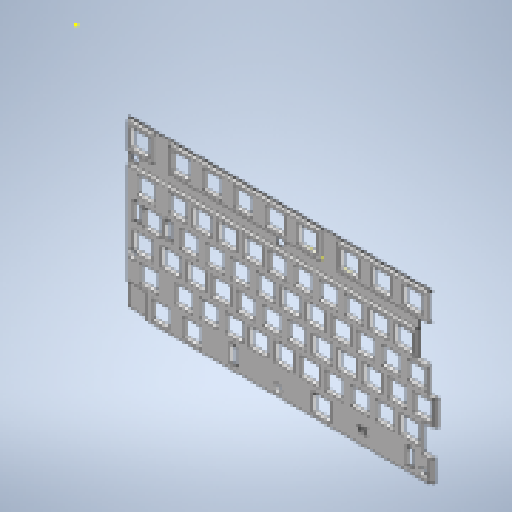
# Autodesk Inventor part: Left Plate
Saved by Autodesk Inventor 2025 (Build 290162000, 162)
## iProperties
Created: 2024-08-20
Part Number: Left Plate
Material: Generic
Document SubType Name: Modeling
Designer: adam
Density: 1 g/cm^3
Appearance: Default
Author: adam
Autodesk Inventor part; units mm, degrees
(part 1 of 2)
ref_plane "YZ Plane" through (0, 0, 0) normal (1, 0, 0) x (0, 1, 0)
ref_plane "XZ Plane" through (0, 0, 0) normal (0, 1, 0) x (-1, 0, 0)
ref_plane "XY Plane" through (0, 0, 0) normal (0, 0, 1) x (1, 0, 0)
sketch "Sketch2" plane through (0, 0, 0) normal (0, 0, 1) x (1, 0, 0)
  line L0 (490, -165) -> (40, -165) projected
  line L1 (490, -40) -> (490, -165) projected
  line L2 (40, -40) -> (490, -40) projected
  line L3 (40, -165) -> (40, -40) projected
  circle A0 centre (62.4608, -160.0704) radius 0.725 projected
  circle A1 centre (69.4608, -161.1204) radius 0.725 projected
  circle A2 centre (66.8608, -155.3704) radius 2.55 projected
  circle A3 centre (86.3368, -160.0704) radius 0.725 projected
  circle A4 centre (93.3368, -161.1204) radius 0.725 projected
  circle A5 centre (90.7368, -155.3704) radius 2.55 projected
  line L4 (118.6501, -160.3704) -> (124.6501, -160.3704) projected
  line L5 (118.6501, -145.3704) -> (118.6501, -160.3704) projected
  line L6 (124.6501, -145.3704) -> (118.6501, -145.3704) projected
  line L7 (124.6501, -160.3704) -> (124.6501, -145.3704) projected
  circle A6 centre (53.5708, -141.0204) radius 0.725 projected
  circle A7 centre (60.5708, -142.0704) radius 0.725 projected
  circle A8 centre (79.7328, -141.0204) radius 0.725 projected
  circle A9 centre (86.7328, -142.0704) radius 0.725 projected
  circle A10 centre (57.9708, -136.3204) radius 2.55 projected
  circle A11 centre (84.1328, -136.3204) radius 2.55 projected
  circle A12 centre (105.7828, -142.0704) radius 0.725 projected
  circle A13 centre (98.7828, -141.0204) radius 0.725 projected
  circle A14 centre (124.8328, -142.0704) radius 0.725 projected
  circle A15 centre (117.8328, -141.0204) radius 0.725 projected
  circle A16 centre (136.8828, -141.0204) radius 0.725 projected
  circle A17 centre (143.8828, -142.0704) radius 0.725 projected
  circle A18 centre (103.1828, -136.3204) radius 2.55 projected
  circle A19 centre (122.2328, -136.3204) radius 2.55 projected
  circle A20 centre (141.2828, -136.3204) radius 2.55 projected
  circle A21 centre (155, -160) radius 1.75 projected
  circle A22 centre (184.0001, -160.0704) radius 0.725 projected
  circle A23 centre (191.0001, -161.1204) radius 0.725 projected
  circle A24 centre (188.4001, -155.3704) radius 2.55 projected
  line L8 (252.1501, -160.3704) -> (258.1501, -160.3704) projected
  line L9 (252.1501, -145.3704) -> (252.1501, -160.3704) projected
  line L10 (258.1501, -145.3704) -> (252.1501, -145.3704) projected
  line L11 (258.1501, -160.3704) -> (258.1501, -145.3704) projected
  circle A25 centre (162.9328, -142.0704) radius 0.725 projected
  circle A26 centre (155.9328, -141.0204) radius 0.725 projected
  circle A27 centre (174.9828, -141.0204) radius 0.725 projected
  circle A28 centre (181.9828, -142.0704) radius 0.725 projected
  circle A29 centre (194.0328, -141.0204) radius 0.725 projected
  circle A30 centre (201.0328, -142.0704) radius 0.725 projected
  circle A31 centre (160.3328, -136.3204) radius 2.55 projected
  circle A32 centre (179.3828, -136.3204) radius 2.55 projected
  circle A33 centre (198.4328, -136.3204) radius 2.55 projected
  circle A34 centre (220.0828, -142.0704) radius 0.725 projected
  circle A35 centre (213.0828, -141.0204) radius 0.725 projected
  circle A36 centre (232.1368, -141.0224) radius 0.725 projected
  circle A37 centre (239.1368, -142.0724) radius 0.725 projected
  circle A38 centre (258.1768, -142.0924) radius 0.725 projected
  circle A39 centre (251.1768, -141.0424) radius 0.725 projected
  circle A40 centre (217.4828, -136.3204) radius 2.55 projected
  circle A41 centre (236.5368, -136.3224) radius 2.55 projected
  circle A42 centre (255.5768, -136.3424) radius 2.55 projected
  circle A43 centre (45, -127) radius 1.75 projected
  circle A44 centre (55.7448, -123.0204) radius 0.725 projected
  circle A45 centre (48.7448, -121.9704) radius 0.725 projected
  circle A46 centre (70.0808, -121.9704) radius 0.725 projected
  circle A47 centre (53.1448, -117.2704) radius 2.55 projected
  circle A48 centre (77.0808, -123.0204) radius 0.725 projected
  circle A49 centre (96.1308, -123.0204) radius 0.725 projected
  circle A50 centre (89.1308, -121.9704) radius 0.725 projected
  circle A51 centre (74.4808, -117.2704) radius 2.55 projected
  circle A52 centre (93.5308, -117.2704) radius 2.55 projected
  circle A53 centre (108.1808, -121.9704) radius 0.725 projected
  circle A54 centre (115.1808, -123.0204) radius 0.725 projected
  circle A55 centre (112.5808, -117.2704) radius 2.55 projected
  circle A56 centre (134.2308, -123.0204) radius 0.725 projected
  circle A57 centre (127.2308, -121.9704) radius 0.725 projected
  circle A58 centre (153.2808, -123.0204) radius 0.725 projected
  circle A59 centre (146.2808, -121.9704) radius 0.725 projected
  circle A60 centre (131.6308, -117.2704) radius 2.55 projected
  circle A61 centre (150.6808, -117.2704) radius 2.55 projected
  circle A62 centre (55.8568, -102.9204) radius 0.725 projected
  circle A63 centre (62.8568, -103.9704) radius 0.725 projected
  circle A64 centre (84.3048, -102.9204) radius 0.725 projected
  circle A65 centre (91.3048, -103.9704) radius 0.725 projected
  circle A66 centre (103.3548, -102.9204) radius 0.725 projected
  circle A67 centre (110.3548, -103.9704) radius 0.725 projected
  circle A68 centre (122.4048, -102.9204) radius 0.725 projected
  circle A69 centre (129.4048, -103.9704) radius 0.725 projected
  circle A70 centre (141.4548, -102.9204) radius 0.725 projected
  circle A71 centre (148.4548, -103.9704) radius 0.725 projected
  circle A72 centre (165.3308, -121.9704) radius 0.725 projected
  circle A73 centre (172.3308, -123.0204) radius 0.725 projected
  circle A74 centre (169.7308, -117.2704) radius 2.55 projected
  circle A75 centre (191.3808, -123.0204) radius 0.725 projected
  circle A76 centre (184.3808, -121.9704) radius 0.725 projected
  circle A77 centre (203.4308, -121.9704) radius 0.725 projected
  circle A78 centre (188.7808, -117.2704) radius 2.55 projected
  circle A79 centre (207.8308, -117.2704) radius 2.55 projected
  circle A80 centre (210.4308, -123.0204) radius 0.725 projected
  circle A81 centre (222.4808, -121.9704) radius 0.725 projected
  circle A82 centre (229.4808, -123.0204) radius 0.725 projected
  circle A83 centre (226.8808, -117.2704) radius 2.55 projected
  circle A84 centre (248.5308, -123.0204) radius 0.725 projected
  circle A85 centre (241.5308, -121.9704) radius 0.725 projected
  circle A86 centre (260.8348, -121.9704) radius 0.725 projected
  circle A87 centre (245.9308, -117.2704) radius 2.55 projected
  circle A88 centre (167.5048, -104.0492) radius 0.725 projected
  circle A89 centre (160.5048, -102.9992) radius 0.725 projected
  circle A90 centre (179.5548, -102.9204) radius 0.725 projected
  circle A91 centre (186.5548, -103.9704) radius 0.725 projected
  circle A92 centre (198.6048, -102.9204) radius 0.725 projected
  circle A93 centre (205.6048, -103.9704) radius 0.725 projected
  circle A94 centre (217.6548, -102.9204) radius 0.725 projected
  circle A95 centre (224.6548, -103.9704) radius 0.725 projected
  circle A96 centre (236.7048, -102.9204) radius 0.725 projected
  circle A97 centre (243.7048, -103.9704) radius 0.725 projected
  circle A98 centre (255.7548, -102.9204) radius 0.725 projected
  circle A99 centre (262.7548, -103.9704) radius 0.725 projected
  circle A100 centre (265, -160) radius 1.75 projected
  circle A101 centre (281.6628, -160.0704) radius 0.725 projected
  circle A102 centre (288.6628, -161.1204) radius 0.725 projected
  circle A103 centre (286.0628, -155.3704) radius 2.55 projected
  circle A104 centre (305.5388, -160.0704) radius 0.725 projected
  circle A105 centre (312.5388, -161.1204) radius 0.725 projected
  circle A106 centre (309.9388, -155.3704) radius 2.55 projected
  circle A107 centre (375, -160) radius 1.75 projected
  circle A108 centre (277.2328, -142.0704) radius 0.725 projected
  circle A109 centre (270.2328, -141.0204) radius 0.725 projected
  circle A110 centre (306.0468, -141.0204) radius 0.725 projected
  circle A111 centre (313.0468, -142.0704) radius 0.725 projected
  circle A112 centre (274.6328, -136.3204) radius 2.55 projected
  circle A113 centre (310.4468, -136.3204) radius 2.55 projected
  line L12 (295.4468, -141.3204) -> (301.4468, -141.3204) projected
  line L13 (295.4468, -126.3204) -> (295.4468, -141.3204) projected
  line L14 (301.4468, -126.3204) -> (295.4468, -126.3204) projected
  line L15 (301.4468, -141.3204) -> (301.4468, -126.3204) projected
  circle A114 centre (357.43, -142.0196) radius 0.725 projected
  circle A115 centre (350.43, -140.9696) radius 0.725 projected
  circle A116 centre (369.48, -140.9696) radius 0.725 projected
  line L16 (319.4468, -141.3204) -> (325.4468, -141.3204) projected
  line L17 (319.4468, -126.3204) -> (319.4468, -141.3204) projected
  line L18 (325.4468, -126.3204) -> (319.4468, -126.3204) projected
  line L19 (325.4468, -141.3204) -> (325.4468, -126.3204) projected
  circle A117 centre (354.83, -136.2696) radius 2.55 projected
  circle A118 centre (373.88, -136.2696) radius 2.55 projected
  circle A119 centre (426.8108, -160.0704) radius 0.725 projected
  circle A120 centre (431.2108, -155.3704) radius 2.55 projected
  line L20 (416.2108, -160.3704) -> (422.2108, -160.3704) projected
  line L21 (416.2108, -145.3704) -> (416.2108, -160.3704) projected
  line L22 (422.2108, -145.3704) -> (416.2108, -145.3704) projected
  line L23 (422.2108, -160.3704) -> (422.2108, -145.3704) projected
  circle A121 centre (433.8108, -161.1204) radius 0.725 projected
  circle A122 centre (455.2588, -160.0704) radius 0.725 projected
  circle A123 centre (462.2588, -161.1204) radius 0.725 projected
  circle A124 centre (459.6588, -155.3704) radius 2.55 projected
  line L24 (468.7088, -160.774) -> (483.7088, -160.774) projected
  line L25 (468.7088, -154.774) -> (468.7088, -160.774) projected
  line L26 (483.7088, -154.774) -> (468.7088, -154.774) projected
  line L27 (483.7088, -160.774) -> (483.7088, -154.774) projected
  line L28 (440.2108, -160.3704) -> (446.2108, -160.3704) projected
  line L29 (440.2108, -145.3704) -> (440.2108, -160.3704) projected
  line L30 (446.2108, -145.3704) -> (440.2108, -145.3704) projected
  line L31 (446.2108, -160.3704) -> (446.2108, -145.3704) projected
  circle A125 centre (483.4088, -150.174) radius 0.725 projected
  circle A126 centre (376.48, -142.0196) radius 0.725 projected
  circle A127 centre (388.53, -140.9696) radius 0.725 projected
  circle A128 centre (395.53, -142.0196) radius 0.725 projected
  circle A129 centre (417.1588, -140.922) radius 0.725 projected
  circle A130 centre (424.1588, -141.972) radius 0.725 projected
  circle A131 centre (392.93, -136.2696) radius 2.55 projected
  circle A132 centre (421.5588, -136.222) radius 2.55 projected
  circle A133 centre (443.2088, -141.972) radius 0.725 projected
  circle A134 centre (436.2088, -140.922) radius 0.725 projected
  circle A135 centre (455.2588, -140.922) radius 0.725 projected
  circle A136 centre (478.7088, -145.774) radius 2.55 projected
  circle A137 centre (462.2588, -141.972) radius 0.725 projected
  circle A138 centre (484.4588, -143.174) radius 0.725 projected
  circle A139 centre (440.6088, -136.222) radius 2.55 projected
  circle A140 centre (459.6588, -136.222) radius 2.55 projected
  line L32 (468.7088, -136.774) -> (483.7088, -136.774) projected
  line L33 (468.7088, -130.774) -> (468.7088, -136.774) projected
  line L34 (483.7088, -130.774) -> (468.7088, -130.774) projected
  line L35 (483.7088, -136.774) -> (483.7088, -130.774) projected
  circle A141 centre (267.8348, -123.0204) radius 0.725 projected
  circle A142 centre (286.8848, -123.0204) radius 0.725 projected
  circle A143 centre (279.8848, -121.9704) radius 0.725 projected
  circle A144 centre (265.2348, -117.2704) radius 2.55 projected
  circle A145 centre (284.2848, -117.2704) radius 2.55 projected
  circle A146 centre (305.9348, -123.0204) radius 0.725 projected
  circle A147 centre (298.9348, -121.9704) radius 0.725 projected
  circle A148 centre (303.3348, -117.2704) radius 2.55 projected
  line L36 (315.6708, -122.8724) -> (330.6708, -122.8724) projected
  line L37 (315.6708, -116.8724) -> (315.6708, -122.8724) projected
  line L38 (330.6708, -116.8724) -> (315.6708, -116.8724) projected
  line L39 (330.6708, -122.8724) -> (330.6708, -116.8724) projected
  circle A149 centre (369.48, -121.9196) radius 0.725 projected
  circle A150 centre (373.88, -117.2196) radius 2.55 projected
  circle A151 centre (274.8048, -102.9204) radius 0.725 projected
  circle A152 centre (281.8048, -103.9704) radius 0.725 projected
  circle A153 centre (293.8548, -102.9204) radius 0.725 projected
  circle A154 centre (300.8548, -103.9704) radius 0.725 projected
  circle A155 centre (329.3458, -112.2974) radius 0.725 projected
  circle A156 centre (324.6458, -107.8974) radius 2.55 projected
  circle A157 centre (330.3958, -105.2974) radius 0.725 projected
  circle A158 centre (376.48, -122.9696) radius 0.725 projected
  circle A159 centre (417.1588, -121.872) radius 0.725 projected
  circle A160 centre (424.1588, -122.922) radius 0.725 projected
  circle A161 centre (421.5588, -117.172) radius 2.55 projected
  circle A162 centre (485, -127) radius 1.75 projected
  circle A163 centre (443.2088, -122.922) radius 0.725 projected
  circle A164 centre (436.2088, -121.872) radius 0.725 projected
  circle A165 centre (455.2588, -121.872) radius 0.725 projected
  circle A166 centre (440.6088, -117.172) radius 2.55 projected
  circle A167 centre (462.2588, -122.922) radius 0.725 projected
  circle A168 centre (481.3088, -122.922) radius 0.725 projected
  circle A169 centre (474.3088, -121.872) radius 0.725 projected
  circle A170 centre (459.6588, -117.172) radius 2.55 projected
  circle A171 centre (478.7088, -117.172) radius 2.55 projected
  circle A172 centre (417.1588, -102.822) radius 0.725 projected
  circle A173 centre (424.1588, -103.872) radius 0.725 projected
  circle A174 centre (436.2088, -102.822) radius 0.725 projected
  circle A175 centre (443.2088, -103.872) radius 0.725 projected
  circle A176 centre (455.2588, -102.822) radius 0.725 projected
  circle A177 centre (462.2588, -103.872) radius 0.725 projected
  circle A178 centre (474.3088, -102.822) radius 0.725 projected
  circle A179 centre (481.3088, -103.872) radius 0.725 projected
  line L40 (45.2568, -103.2204) -> (51.2568, -103.2204) projected
  line L41 (45.2568, -88.2204) -> (45.2568, -103.2204) projected
  line L42 (51.2568, -88.2204) -> (45.2568, -88.2204) projected
  line L43 (51.2568, -103.2204) -> (51.2568, -88.2204) projected
  circle A180 centre (60.2568, -98.2204) radius 2.55 projected
  line L44 (69.2568, -103.2204) -> (75.2568, -103.2204) projected
  line L45 (69.2568, -88.2204) -> (69.2568, -103.2204) projected
  line L46 (75.2568, -88.2204) -> (69.2568, -88.2204) projected
  line L47 (75.2568, -103.2204) -> (75.2568, -88.2204) projected
  circle A181 centre (88.7048, -98.2204) radius 2.55 projected
  circle A182 centre (107.7548, -98.2204) radius 2.55 projected
  circle A183 centre (126.8048, -98.2204) radius 2.55 projected
  circle A184 centre (145.8548, -98.2204) radius 2.55 projected
  circle A185 centre (51.1288, -83.8704) radius 0.725 projected
  circle A186 centre (58.1288, -84.9204) radius 0.725 projected
  circle A187 centre (74.9068, -83.8704) radius 0.725 projected
  circle A188 centre (81.9068, -84.9204) radius 0.725 projected
  circle A189 centre (93.9568, -83.8704) radius 0.725 projected
  circle A190 centre (55.5288, -79.1704) radius 2.55 projected
  circle A191 centre (79.3068, -79.1704) radius 2.55 projected
  circle A192 centre (98.3568, -79.1704) radius 2.55 projected
  circle A193 centre (100.9568, -84.9204) radius 0.725 projected
  circle A194 centre (113.0068, -83.8704) radius 0.725 projected
  circle A195 centre (120.0068, -84.9204) radius 0.725 projected
  circle A196 centre (132.0568, -83.8704) radius 0.725 projected
  circle A197 centre (139.0568, -84.9204) radius 0.725 projected
  circle A198 centre (151.1068, -83.8704) radius 0.725 projected
  circle A199 centre (117.4068, -79.1704) radius 2.55 projected
  circle A200 centre (136.4568, -79.1704) radius 2.55 projected
  circle A201 centre (164.9048, -98.2992) radius 2.55 projected
  circle A202 centre (183.9548, -98.2204) radius 2.55 projected
  circle A203 centre (203.0048, -98.2204) radius 2.55 projected
  circle A204 centre (222.0548, -98.2204) radius 2.55 projected
  circle A205 centre (241.1048, -98.2204) radius 2.55 projected
  circle A206 centre (260.1548, -98.2204) radius 2.55 projected
  circle A207 centre (158.1068, -84.9204) radius 0.725 projected
  circle A208 centre (170.1568, -83.8704) radius 0.725 projected
  circle A209 centre (177.1568, -84.9204) radius 0.725 projected
  circle A210 centre (189.2068, -83.8704) radius 0.725 projected
  circle A211 centre (196.2068, -84.9204) radius 0.725 projected
  circle A212 centre (208.2568, -83.8704) radius 0.725 projected
  circle A213 centre (155.5068, -79.1704) radius 2.55 projected
  circle A214 centre (174.5568, -79.1704) radius 2.55 projected
  circle A215 centre (193.6068, -79.1704) radius 2.55 projected
  circle A216 centre (215.2568, -84.9204) radius 0.725 projected
  circle A217 centre (227.3068, -83.8704) radius 0.725 projected
  circle A218 centre (234.3068, -84.9204) radius 0.725 projected
  circle A219 centre (246.3568, -83.8704) radius 0.725 projected
  circle A220 centre (253.3568, -84.9204) radius 0.725 projected
  circle A221 centre (212.6568, -79.1704) radius 2.55 projected
  circle A222 centre (231.7068, -79.1704) radius 2.55 projected
  circle A223 centre (250.7568, -79.1704) radius 2.55 projected
  circle A224 centre (45, -64.8616) radius 1.75 projected
  circle A225 centre (50.8588, -50.6116) radius 2.55 projected
  circle A226 centre (81.9072, -50.3984) radius 2.55 projected
  circle A227 centre (48.2588, -44.8616) radius 0.725 projected
  circle A228 centre (55.2588, -45.9116) radius 0.725 projected
  circle A229 centre (79.3072, -44.6484) radius 0.725 projected
  circle A230 centre (86.3072, -45.6984) radius 0.725 projected
  circle A231 centre (105.7228, -50.5136) radius 2.55 projected
  circle A232 centre (129.5988, -50.5416) radius 2.55 projected
  circle A233 centre (153.4748, -50.5136) radius 2.55 projected
  circle A234 centre (103.1228, -44.7636) radius 0.725 projected
  circle A235 centre (110.1228, -45.8136) radius 0.725 projected
  circle A236 centre (126.9988, -44.7916) radius 0.725 projected
  circle A237 centre (133.9988, -45.8416) radius 0.725 projected
  circle A238 centre (150.8748, -44.7636) radius 0.725 projected
  circle A239 centre (155, -64.8616) radius 1.75 projected
  circle A240 centre (175.2648, -63.1601) radius 0.425 projected
  circle A241 centre (177.7648, -63.1601) radius 0.425 projected
  circle A242 centre (180.2648, -63.1601) radius 0.425 projected
  circle A243 centre (174.0148, -60.6601) radius 0.425 projected
  circle A244 centre (176.5148, -60.6601) radius 0.425 projected
  circle A245 centre (179.0148, -60.6601) radius 0.425 projected
  circle A246 centre (181.5148, -60.6601) radius 0.425 projected
  circle A247 centre (182.7648, -63.1601) radius 0.425 projected
  circle A248 centre (185.2648, -63.1601) radius 0.425 projected
  circle A249 centre (187.7648, -63.1601) radius 0.425 projected
  circle A250 centre (190.2648, -63.1601) radius 0.425 projected
  circle A251 centre (192.7648, -63.1601) radius 0.425 projected
  circle A252 centre (195.2648, -63.1601) radius 0.425 projected
  circle A253 centre (197.7648, -63.1601) radius 0.425 projected
  circle A254 centre (200.2648, -63.1601) radius 0.425 projected
  circle A255 centre (202.7648, -63.1601) radius 0.425 projected
  circle A256 centre (205.2648, -63.1601) radius 0.425 projected
  circle A257 centre (207.7648, -63.1601) radius 0.425 projected
  circle A258 centre (184.0148, -60.6601) radius 0.425 projected
  circle A259 centre (186.5148, -60.6601) radius 0.425 projected
  circle A260 centre (189.0148, -60.6601) radius 0.425 projected
  circle A261 centre (191.5148, -60.6601) radius 0.425 projected
  circle A262 centre (194.0148, -60.6601) radius 0.425 projected
  circle A263 centre (196.5148, -60.6601) radius 0.425 projected
  circle A264 centre (199.0148, -60.6601) radius 0.425 projected
  circle A265 centre (201.5148, -60.6601) radius 0.425 projected
  circle A266 centre (204.0148, -60.6601) radius 0.425 projected
  circle A267 centre (206.5148, -60.6601) radius 0.425 projected
  circle A268 centre (209.0148, -60.6601) radius 0.425 projected
  circle A269 centre (210.2648, -63.1601) radius 0.425 projected
  circle A270 centre (212.7648, -63.1601) radius 0.425 projected
  circle A271 centre (211.5148, -60.6601) radius 0.425 projected
  circle A272 centre (177.3508, -50.5136) radius 2.55 projected
  circle A273 centre (157.8748, -45.8136) radius 0.725 projected
  circle A274 centre (174.7508, -44.7636) radius 0.725 projected
  circle A275 centre (181.7508, -45.8136) radius 0.725 projected
  circle A276 centre (207.2568, -44.7636) radius 0.725 projected
  circle A277 centre (209.8568, -50.5136) radius 2.55 projected
  circle A278 centre (233.7388, -50.5136) radius 2.55 projected
  circle A279 centre (257.6148, -50.5136) radius 2.55 projected
  circle A280 centre (214.2568, -45.8136) radius 0.725 projected
  circle A281 centre (231.1388, -44.7636) radius 0.725 projected
  circle A282 centre (238.1388, -45.8136) radius 0.725 projected
  circle A283 centre (255.0148, -44.7636) radius 0.725 projected
  circle A284 centre (262.0148, -45.8136) radius 0.725 projected
  circle A285 centre (279.2048, -98.2204) radius 2.55 projected
  circle A286 centre (298.2548, -98.2204) radius 2.55 projected
  line L48 (315.6708, -98.8724) -> (330.6708, -98.8724) projected
  line L49 (315.6708, -92.8724) -> (315.6708, -98.8724) projected
  line L50 (330.6708, -92.8724) -> (315.6708, -92.8724) projected
  line L51 (330.6708, -98.8724) -> (330.6708, -92.8724) projected
  circle A287 centre (265.4068, -83.8704) radius 0.725 projected
  circle A288 centre (272.4068, -84.9204) radius 0.725 projected
  circle A289 centre (284.4568, -83.8704) radius 0.725 projected
  circle A290 centre (291.4568, -84.9204) radius 0.725 projected
  circle A291 centre (303.5068, -83.8704) radius 0.725 projected
  circle A292 centre (310.5068, -84.9204) radius 0.725 projected
  circle A293 centre (269.8068, -79.1704) radius 2.55 projected
  circle A294 centre (288.8568, -79.1704) radius 2.55 projected
  circle A295 centre (307.9068, -79.1704) radius 2.55 projected
  circle A296 centre (322.5568, -83.8704) radius 0.725 projected
  circle A297 centre (329.5568, -84.9204) radius 0.725 projected
  circle A298 centre (355.158, -83.8056) radius 0.725 projected
  circle A299 centre (362.158, -84.8556) radius 0.725 projected
  circle A300 centre (326.9568, -79.1704) radius 2.55 projected
  circle A301 centre (359.558, -79.1056) radius 2.55 projected
  circle A302 centre (421.5588, -98.122) radius 2.55 projected
  circle A303 centre (440.6088, -98.122) radius 2.55 projected
  circle A304 centre (459.6588, -98.122) radius 2.55 projected
  circle A305 centre (478.7088, -98.122) radius 2.55 projected
  circle A306 centre (383.754, -83.8056) radius 0.725 projected
  circle A307 centre (390.754, -84.8556) radius 0.725 projected
  circle A308 centre (417.1588, -83.772) radius 0.725 projected
  circle A309 centre (424.1588, -84.822) radius 0.725 projected
  circle A310 centre (388.154, -79.1056) radius 2.55 projected
  circle A311 centre (421.5588, -79.072) radius 2.55 projected
  circle A312 centre (436.2088, -83.772) radius 0.725 projected
  circle A313 centre (443.2088, -84.822) radius 0.725 projected
  circle A314 centre (455.2588, -83.772) radius 0.725 projected
  circle A315 centre (462.2588, -84.822) radius 0.725 projected
  circle A316 centre (474.3088, -83.772) radius 0.725 projected
  circle A317 centre (481.3088, -84.822) radius 0.725 projected
  circle A318 centre (440.6088, -79.072) radius 2.55 projected
  circle A319 centre (459.6588, -79.072) radius 2.55 projected
  circle A320 centre (478.7088, -79.072) radius 2.55 projected
  circle A321 centre (265, -64.8616) radius 1.75 projected
  circle A322 centre (375, -64.8616) radius 1.75 projected
  circle A323 centre (281.4908, -50.5136) radius 2.55 projected
  circle A324 centre (305.3668, -50.5136) radius 2.55 projected
  circle A325 centre (278.8908, -44.7636) radius 0.725 projected
  circle A326 centre (285.8908, -45.8136) radius 0.725 projected
  circle A327 centre (302.7668, -44.7636) radius 0.725 projected
  circle A328 centre (309.7668, -45.8136) radius 0.725 projected
  circle A329 centre (333.3668, -48.0136) radius 5 projected
  circle A330 centre (485, -64.8616) radius 1.75 projected
  circle A331 centre (408.3668, -48.0136) radius 5 projected
  circle A332 centre (453.2088, -50.322) radius 5 projected
  circle A333 centre (481.2088, -50.322) radius 5 projected
  circle A334 centre (432.68, -43) radius 0.5 projected
  circle A335 centre (435.22, -43) radius 0.5 projected
  circle A336 centre (437.76, -43) radius 0.5 projected
  circle A337 centre (440.3, -43) radius 0.5 projected
  line L52 (172.0148, -58.6601) -> (214.7648, -58.6601)
  line L53 (214.7648, -58.6601) -> (214.7648, -65.1601)
  line L54 (214.7648, -65.1601) -> (172.0148, -65.1601)
  line L55 (172.0148, -65.1601) -> (172.0148, -58.6601)
  line L56 (272.1064, -165) -> (272.1064, -148.1602) construction
  line L57 (272.1064, -148.1602) -> (265.1048, -148.1602) construction
  line L58 (265.1048, -148.1602) -> (265.1048, -126.7954) construction
  line L59 (265.1048, -126.7954) -> (274.7598, -126.7954) construction
  line L60 (274.7598, -126.7954) -> (274.7598, -107.7454) construction
  line L61 (274.7598, -107.7454) -> (269.6798, -107.7454) construction
  line L62 (269.6798, -107.7454) -> (269.6798, -88.6954) construction
  line L63 (269.6798, -88.6954) -> (260.2818, -88.6954) construction
  line L64 (260.2818, -88.6954) -> (260.2818, -61.0161) construction
  line L65 (260.2818, -61.0161) -> (269.5528, -61.0161) construction
  line L66 (269.5528, -61.0161) -> (269.5528, -40) construction
  line L67 (257.6148, -50.5136) -> (269.5528, -50.5136) construction
  line L68 (269.5528, -50.5136) -> (281.4908, -50.5136) construction
  line L69 (269.8068, -79.1704) -> (260.2818, -79.1704) construction
  line L70 (250.7568, -79.1704) -> (260.2818, -79.1704) construction
  line L71 (260.1548, -98.2204) -> (269.6798, -98.2204) construction
  line L72 (279.2048, -98.2204) -> (269.6798, -98.2204) construction
  line L73 (265.2348, -117.2704) -> (274.7598, -117.2704) construction
  line L74 (284.2848, -117.2704) -> (274.7598, -117.2704) construction
  line L75 (274.6328, -136.3204) -> (265.1048, -136.3204) construction
  line L76 (255.5768, -136.3424) -> (265.1048, -136.3204) construction
  line L77 (286.0628, -155.3704) -> (272.1064, -155.4026) construction
  line L78 (258.1501, -155.4349) -> (272.1064, -155.4026) construction
  line L79 (269.8688, -136.3204) -> (269.8688, -126.7954) construction
  line L80 (269.8688, -126.7954) -> (269.8688, -117.2704) construction
  line L81 (271.6818, -117.2704) -> (271.6818, -107.7454) construction
  line L82 (271.6818, -107.7454) -> (271.6818, -98.2204) construction
  line L83 (263.5838, -98.2204) -> (263.5838, -88.6954) construction
  line L84 (263.5838, -88.6954) -> (263.5838, -79.1704) construction
  line L85 (250.6123, -43.5111) -> (264.6173, -43.5111)
  line L86 (264.6173, -43.5111) -> (264.6173, -57.5161)
  line L87 (264.6173, -57.5161) -> (250.6123, -57.5161)
  line L88 (250.6123, -57.5161) -> (250.6123, -43.5111)
  line L89 (250.6123, -43.5111) -> (264.6173, -57.5161) construction
  line L90 (264.6173, -43.5111) -> (250.6123, -57.5161) construction
  line L91 (226.7363, -43.5111) -> (240.7413, -43.5111)
  line L92 (240.7413, -43.5111) -> (240.7413, -57.5161)
  line L93 (240.7413, -57.5161) -> (226.7363, -57.5161)
  line L94 (226.7363, -57.5161) -> (226.7363, -43.5111)
  line L95 (226.7363, -43.5111) -> (240.7413, -57.5161) construction
  line L96 (240.7413, -43.5111) -> (226.7363, -57.5161) construction
  line L97 (202.8543, -43.5111) -> (216.8593, -43.5111)
  line L98 (216.8593, -43.5111) -> (216.8593, -57.5161)
  line L99 (216.8593, -57.5161) -> (202.8543, -57.5161)
  line L100 (202.8543, -57.5161) -> (202.8543, -43.5111)
  line L101 (202.8543, -43.5111) -> (216.8593, -57.5161) construction
  line L102 (216.8593, -43.5111) -> (202.8543, -57.5161) construction
  line L103 (170.3483, -43.5111) -> (184.3533, -43.5111)
  line L104 (184.3533, -43.5111) -> (184.3533, -57.5161)
  line L105 (184.3533, -57.5161) -> (170.3483, -57.5161)
  line L106 (170.3483, -57.5161) -> (170.3483, -43.5111)
  line L107 (170.3483, -43.5111) -> (184.3533, -57.5161) construction
  line L108 (184.3533, -43.5111) -> (170.3483, -57.5161) construction
  line L109 (146.4723, -43.5111) -> (160.4773, -43.5111)
  line L110 (160.4773, -43.5111) -> (160.4773, -57.5161)
  line L111 (160.4773, -57.5161) -> (146.4723, -57.5161)
  line L112 (146.4723, -57.5161) -> (146.4723, -43.5111)
  line L113 (146.4723, -43.5111) -> (160.4773, -57.5161) construction
  line L114 (160.4773, -43.5111) -> (146.4723, -57.5161) construction
  line L115 (122.5963, -43.5391) -> (136.6013, -43.5391)
  line L116 (136.6013, -43.5391) -> (136.6013, -57.5441)
  line L117 (136.6013, -57.5441) -> (122.5963, -57.5441)
  line L118 (122.5963, -57.5441) -> (122.5963, -43.5391)
  line L119 (122.5963, -43.5391) -> (136.6013, -57.5441) construction
  line L120 (136.6013, -43.5391) -> (122.5963, -57.5441) construction
  line L121 (98.7203, -43.5111) -> (112.7253, -43.5111)
  line L122 (112.7253, -43.5111) -> (112.7253, -57.5161)
  line L123 (112.7253, -57.5161) -> (98.7203, -57.5161)
  line L124 (98.7203, -57.5161) -> (98.7203, -43.5111)
  line L125 (98.7203, -43.5111) -> (112.7253, -57.5161) construction
  line L126 (112.7253, -43.5111) -> (98.7203, -57.5161) construction
  line L127 (74.9047, -43.3959) -> (88.9097, -43.3959)
  line L128 (88.9097, -43.3959) -> (88.9097, -57.4009)
  line L129 (88.9097, -57.4009) -> (74.9047, -57.4009)
  line L130 (74.9047, -57.4009) -> (74.9047, -43.3959)
  line L131 (74.9047, -43.3959) -> (88.9097, -57.4009) construction
  line L132 (88.9097, -43.3959) -> (74.9047, -57.4009) construction
  line L133 (43.8563, -43.6091) -> (57.8613, -43.6091)
  line L134 (57.8613, -43.6091) -> (57.8613, -57.6141)
  line L135 (57.8613, -57.6141) -> (43.8563, -57.6141)
  line L136 (43.8563, -57.6141) -> (43.8563, -43.6091)
  line L137 (43.8563, -43.6091) -> (57.8613, -57.6141) construction
  line L138 (57.8613, -43.6091) -> (43.8563, -57.6141) construction
  line L139 (48.5263, -72.1679) -> (62.5313, -72.1679)
  line L140 (62.5313, -72.1679) -> (62.5313, -86.1729)
  line L141 (62.5313, -86.1729) -> (48.5263, -86.1729)
  line L142 (48.5263, -86.1729) -> (48.5263, -72.1679)
  line L143 (48.5263, -72.1679) -> (62.5313, -86.1729) construction
  line L144 (62.5313, -72.1679) -> (48.5263, -86.1729) construction
  line L145 (72.3043, -72.1679) -> (86.3093, -72.1679)
  line L146 (86.3093, -72.1679) -> (86.3093, -86.1729)
  line L147 (86.3093, -86.1729) -> (72.3043, -86.1729)
  line L148 (72.3043, -86.1729) -> (72.3043, -72.1679)
  line L149 (72.3043, -72.1679) -> (86.3093, -86.1729) construction
  line L150 (86.3093, -72.1679) -> (72.3043, -86.1729) construction
  line L151 (91.3543, -72.1679) -> (105.3593, -72.1679)
  line L152 (105.3593, -72.1679) -> (105.3593, -86.1729)
  line L153 (105.3593, -86.1729) -> (91.3543, -86.1729)
  line L154 (91.3543, -86.1729) -> (91.3543, -72.1679)
  line L155 (91.3543, -72.1679) -> (105.3593, -86.1729) construction
  line L156 (105.3593, -72.1679) -> (91.3543, -86.1729) construction
  line L157 (110.4043, -72.1679) -> (124.4093, -72.1679)
  line L158 (124.4093, -72.1679) -> (124.4093, -86.1729)
  line L159 (124.4093, -86.1729) -> (110.4043, -86.1729)
  line L160 (110.4043, -86.1729) -> (110.4043, -72.1679)
  line L161 (110.4043, -72.1679) -> (124.4093, -86.1729) construction
  line L162 (124.4093, -72.1679) -> (110.4043, -86.1729) construction
  line L163 (129.4543, -72.1679) -> (143.4593, -72.1679)
  line L164 (143.4593, -72.1679) -> (143.4593, -86.1729)
  line L165 (143.4593, -86.1729) -> (129.4543, -86.1729)
  line L166 (129.4543, -86.1729) -> (129.4543, -72.1679)
  line L167 (129.4543, -72.1679) -> (143.4593, -86.1729) construction
  line L168 (143.4593, -72.1679) -> (129.4543, -86.1729) construction
  line L169 (148.5043, -72.1679) -> (162.5093, -72.1679)
  line L170 (162.5093, -72.1679) -> (162.5093, -86.1729)
  line L171 (162.5093, -86.1729) -> (148.5043, -86.1729)
  line L172 (148.5043, -86.1729) -> (148.5043, -72.1679)
  line L173 (148.5043, -72.1679) -> (162.5093, -86.1729) construction
  line L174 (162.5093, -72.1679) -> (148.5043, -86.1729) construction
  line L175 (167.5543, -72.1679) -> (181.5593, -72.1679)
  line L176 (181.5593, -72.1679) -> (181.5593, -86.1729)
  line L177 (181.5593, -86.1729) -> (167.5543, -86.1729)
  line L178 (167.5543, -86.1729) -> (167.5543, -72.1679)
  line L179 (167.5543, -72.1679) -> (181.5593, -86.1729) construction
  line L180 (181.5593, -72.1679) -> (167.5543, -86.1729) construction
  line L181 (53.2543, -91.2179) -> (67.2593, -91.2179)
  line L182 (67.2593, -91.2179) -> (67.2593, -105.2229)
  line L183 (67.2593, -105.2229) -> (53.2543, -105.2229)
  line L184 (53.2543, -105.2229) -> (53.2543, -91.2179)
  line L185 (53.2543, -91.2179) -> (67.2593, -105.2229) construction
  line L186 (67.2593, -91.2179) -> (53.2543, -105.2229) construction
  line L187 (186.6043, -72.1679) -> (200.6093, -72.1679)
  line L188 (200.6093, -72.1679) -> (200.6093, -86.1729)
  line L189 (200.6093, -86.1729) -> (186.6043, -86.1729)
  line L190 (186.6043, -86.1729) -> (186.6043, -72.1679)
  line L191 (186.6043, -72.1679) -> (200.6093, -86.1729) construction
  line L192 (200.6093, -72.1679) -> (186.6043, -86.1729) construction
  line L193 (205.6543, -72.1679) -> (219.6593, -72.1679)
  line L194 (219.6593, -72.1679) -> (219.6593, -86.1729)
  line L195 (219.6593, -86.1729) -> (205.6543, -86.1729)
  line L196 (205.6543, -86.1729) -> (205.6543, -72.1679)
  line L197 (205.6543, -72.1679) -> (219.6593, -86.1729) construction
  line L198 (219.6593, -72.1679) -> (205.6543, -86.1729) construction
  line L199 (224.7043, -72.1679) -> (238.7093, -72.1679)
  line L200 (238.7093, -72.1679) -> (238.7093, -86.1729)
  line L201 (238.7093, -86.1729) -> (224.7043, -86.1729)
  line L202 (224.7043, -86.1729) -> (224.7043, -72.1679)
  line L203 (224.7043, -72.1679) -> (238.7093, -86.1729) construction
  line L204 (238.7093, -72.1679) -> (224.7043, -86.1729) construction
  line L205 (243.7543, -72.1679) -> (257.7593, -72.1679)
  line L206 (257.7593, -72.1679) -> (257.7593, -86.1729)
  line L207 (257.7593, -86.1729) -> (243.7543, -86.1729)
  line L208 (243.7543, -86.1729) -> (243.7543, -72.1679)
  line L209 (243.7543, -72.1679) -> (257.7593, -86.1729) construction
  line L210 (257.7593, -72.1679) -> (243.7543, -86.1729) construction
  line L211 (253.1523, -91.2179) -> (267.1573, -91.2179)
  line L212 (267.1573, -91.2179) -> (267.1573, -105.2229)
  line L213 (267.1573, -105.2229) -> (253.1523, -105.2229)
  line L214 (253.1523, -105.2229) -> (253.1523, -91.2179)
  line L215 (253.1523, -91.2179) -> (267.1573, -105.2229) construction
  line L216 (267.1573, -91.2179) -> (253.1523, -105.2229) construction
  line L217 (234.1023, -91.2179) -> (248.1073, -91.2179)
  line L218 (248.1073, -91.2179) -> (248.1073, -105.2229)
  line L219 (248.1073, -105.2229) -> (234.1023, -105.2229)
  line L220 (234.1023, -105.2229) -> (234.1023, -91.2179)
  line L221 (234.1023, -91.2179) -> (248.1073, -105.2229) construction
  line L222 (248.1073, -91.2179) -> (234.1023, -105.2229) construction
  line L223 (215.0523, -91.2179) -> (229.0573, -91.2179)
  line L224 (229.0573, -91.2179) -> (229.0573, -105.2229)
  line L225 (229.0573, -105.2229) -> (215.0523, -105.2229)
  line L226 (215.0523, -105.2229) -> (215.0523, -91.2179)
  line L227 (215.0523, -91.2179) -> (229.0573, -105.2229) construction
  line L228 (229.0573, -91.2179) -> (215.0523, -105.2229) construction
  line L229 (196.0023, -91.2179) -> (210.0073, -91.2179)
  line L230 (210.0073, -91.2179) -> (210.0073, -105.2229)
  line L231 (210.0073, -105.2229) -> (196.0023, -105.2229)
  line L232 (196.0023, -105.2229) -> (196.0023, -91.2179)
  line L233 (196.0023, -91.2179) -> (210.0073, -105.2229) construction
  line L234 (210.0073, -91.2179) -> (196.0023, -105.2229) construction
  line L235 (176.9523, -91.2179) -> (190.9573, -91.2179)
  line L236 (190.9573, -91.2179) -> (190.9573, -105.2229)
  line L237 (190.9573, -105.2229) -> (176.9523, -105.2229)
  line L238 (176.9523, -105.2229) -> (176.9523, -91.2179)
  line L239 (176.9523, -91.2179) -> (190.9573, -105.2229) construction
  line L240 (190.9573, -91.2179) -> (176.9523, -105.2229) construction
  line L241 (157.9023, -91.2967) -> (171.9073, -91.2967)
  line L242 (171.9073, -91.2967) -> (171.9073, -105.3017)
  line L243 (171.9073, -105.3017) -> (157.9023, -105.3017)
  line L244 (157.9023, -105.3017) -> (157.9023, -91.2967)
  line L245 (157.9023, -91.2967) -> (171.9073, -105.3017) construction
  line L246 (171.9073, -91.2967) -> (157.9023, -105.3017) construction
  line L247 (138.8523, -91.2179) -> (152.8573, -91.2179)
  line L248 (152.8573, -91.2179) -> (152.8573, -105.2229)
  line L249 (152.8573, -105.2229) -> (138.8523, -105.2229)
  line L250 (138.8523, -105.2229) -> (138.8523, -91.2179)
  line L251 (138.8523, -91.2179) -> (152.8573, -105.2229) construction
  line L252 (152.8573, -91.2179) -> (138.8523, -105.2229) construction
  line L253 (119.8023, -91.2179) -> (133.8073, -91.2179)
  line L254 (133.8073, -91.2179) -> (133.8073, -105.2229)
  line L255 (133.8073, -105.2229) -> (119.8023, -105.2229)
  line L256 (119.8023, -105.2229) -> (119.8023, -91.2179)
  line L257 (119.8023, -91.2179) -> (133.8073, -105.2229) construction
  line L258 (133.8073, -91.2179) -> (119.8023, -105.2229) construction
  line L259 (100.7523, -91.2179) -> (114.7573, -91.2179)
  line L260 (114.7573, -91.2179) -> (114.7573, -105.2229)
  line L261 (114.7573, -105.2229) -> (100.7523, -105.2229)
  line L262 (100.7523, -105.2229) -> (100.7523, -91.2179)
  line L263 (100.7523, -91.2179) -> (114.7573, -105.2229) construction
  line L264 (114.7573, -91.2179) -> (100.7523, -105.2229) construction
  line L265 (81.7023, -91.2179) -> (95.7073, -91.2179)
  line L266 (95.7073, -91.2179) -> (95.7073, -105.2229)
  line L267 (95.7073, -105.2229) -> (81.7023, -105.2229)
  line L268 (81.7023, -105.2229) -> (81.7023, -91.2179)
  line L269 (81.7023, -91.2179) -> (95.7073, -105.2229) construction
  line L270 (95.7073, -91.2179) -> (81.7023, -105.2229) construction
  line L271 (46.1423, -110.2679) -> (60.1473, -110.2679)
  line L272 (60.1473, -110.2679) -> (60.1473, -124.2729)
  line L273 (60.1473, -124.2729) -> (46.1423, -124.2729)
  line L274 (46.1423, -124.2729) -> (46.1423, -110.2679)
  line L275 (46.1423, -110.2679) -> (60.1473, -124.2729) construction
  line L276 (60.1473, -110.2679) -> (46.1423, -124.2729) construction
  line L277 (67.4783, -110.2679) -> (81.4833, -110.2679)
  line L278 (81.4833, -110.2679) -> (81.4833, -124.2729)
  line L279 (81.4833, -124.2729) -> (67.4783, -124.2729)
  line L280 (67.4783, -124.2729) -> (67.4783, -110.2679)
  line L281 (67.4783, -110.2679) -> (81.4833, -124.2729) construction
  line L282 (81.4833, -110.2679) -> (67.4783, -124.2729) construction
  line L283 (86.5283, -110.2679) -> (100.5333, -110.2679)
  line L284 (100.5333, -110.2679) -> (100.5333, -124.2729)
  line L285 (100.5333, -124.2729) -> (86.5283, -124.2729)
  line L286 (86.5283, -124.2729) -> (86.5283, -110.2679)
  line L287 (86.5283, -110.2679) -> (100.5333, -124.2729) construction
  line L288 (100.5333, -110.2679) -> (86.5283, -124.2729) construction
  line L289 (105.5783, -110.2679) -> (119.5833, -110.2679)
  line L290 (119.5833, -110.2679) -> (119.5833, -124.2729)
  line L291 (119.5833, -124.2729) -> (105.5783, -124.2729)
  line L292 (105.5783, -124.2729) -> (105.5783, -110.2679)
  line L293 (105.5783, -110.2679) -> (119.5833, -124.2729) construction
  line L294 (119.5833, -110.2679) -> (105.5783, -124.2729) construction
  line L295 (124.6283, -110.2679) -> (138.6333, -110.2679)
  line L296 (138.6333, -110.2679) -> (138.6333, -124.2729)
  line L297 (138.6333, -124.2729) -> (124.6283, -124.2729)
  line L298 (124.6283, -124.2729) -> (124.6283, -110.2679)
  line L299 (124.6283, -110.2679) -> (138.6333, -124.2729) construction
  line L300 (138.6333, -110.2679) -> (124.6283, -124.2729) construction
  line L301 (143.6783, -110.2679) -> (157.6833, -110.2679)
  line L302 (157.6833, -110.2679) -> (157.6833, -124.2729)
  line L303 (157.6833, -124.2729) -> (143.6783, -124.2729)
  line L304 (143.6783, -124.2729) -> (143.6783, -110.2679)
  line L305 (143.6783, -110.2679) -> (157.6833, -124.2729) construction
  line L306 (157.6833, -110.2679) -> (143.6783, -124.2729) construction
  line L307 (162.7283, -110.2679) -> (176.7333, -110.2679)
  line L308 (176.7333, -110.2679) -> (176.7333, -124.2729)
  line L309 (176.7333, -124.2729) -> (162.7283, -124.2729)
  line L310 (162.7283, -124.2729) -> (162.7283, -110.2679)
  line L311 (162.7283, -110.2679) -> (176.7333, -124.2729) construction
  line L312 (176.7333, -110.2679) -> (162.7283, -124.2729) construction
  line L313 (181.7783, -110.2679) -> (195.7833, -110.2679)
  line L314 (195.7833, -110.2679) -> (195.7833, -124.2729)
  line L315 (195.7833, -124.2729) -> (181.7783, -124.2729)
  line L316 (181.7783, -124.2729) -> (181.7783, -110.2679)
  line L317 (181.7783, -110.2679) -> (195.7833, -124.2729) construction
  line L318 (195.7833, -110.2679) -> (181.7783, -124.2729) construction
  line L319 (200.8283, -110.2679) -> (214.8333, -110.2679)
  line L320 (214.8333, -110.2679) -> (214.8333, -124.2729)
  line L321 (214.8333, -124.2729) -> (200.8283, -124.2729)
  line L322 (200.8283, -124.2729) -> (200.8283, -110.2679)
  line L323 (200.8283, -110.2679) -> (214.8333, -124.2729) construction
  line L324 (214.8333, -110.2679) -> (200.8283, -124.2729) construction
  line L325 (219.8783, -110.2679) -> (233.8833, -110.2679)
  line L326 (233.8833, -110.2679) -> (233.8833, -124.2729)
  line L327 (233.8833, -124.2729) -> (219.8783, -124.2729)
  line L328 (219.8783, -124.2729) -> (219.8783, -110.2679)
  line L329 (219.8783, -110.2679) -> (233.8833, -124.2729) construction
  line L330 (233.8833, -110.2679) -> (219.8783, -124.2729) construction
  line L331 (238.9283, -110.2679) -> (252.9333, -110.2679)
  line L332 (252.9333, -110.2679) -> (252.9333, -124.2729)
  line L333 (252.9333, -124.2729) -> (238.9283, -124.2729)
  line L334 (238.9283, -124.2729) -> (238.9283, -110.2679)
  line L335 (238.9283, -110.2679) -> (252.9333, -124.2729) construction
  line L336 (252.9333, -110.2679) -> (238.9283, -124.2729) construction
  line L337 (258.2323, -110.2679) -> (272.2373, -110.2679)
  line L338 (272.2373, -110.2679) -> (272.2373, -124.2729)
  line L339 (272.2373, -124.2729) -> (258.2323, -124.2729)
  line L340 (258.2323, -124.2729) -> (258.2323, -110.2679)
  line L341 (258.2323, -110.2679) -> (272.2373, -124.2729) construction
  line L342 (272.2373, -110.2679) -> (258.2323, -124.2729) construction
  line L343 (248.5743, -129.3399) -> (262.5793, -129.3399)
  line L344 (262.5793, -129.3399) -> (262.5793, -143.3449)
  line L345 (262.5793, -143.3449) -> (248.5743, -143.3449)
  line L346 (248.5743, -143.3449) -> (248.5743, -129.3399)
  line L347 (248.5743, -129.3399) -> (262.5793, -143.3449) construction
  line L348 (262.5793, -129.3399) -> (248.5743, -143.3449) construction
  line L349 (229.5343, -129.3199) -> (243.5393, -129.3199)
  line L350 (243.5393, -129.3199) -> (243.5393, -143.3249)
  line L351 (243.5393, -143.3249) -> (229.5343, -143.3249)
  line L352 (229.5343, -143.3249) -> (229.5343, -129.3199)
  line L353 (229.5343, -129.3199) -> (243.5393, -143.3249) construction
  line L354 (243.5393, -129.3199) -> (229.5343, -143.3249) construction
  line L355 (210.4803, -129.3179) -> (224.4853, -129.3179)
  line L356 (224.4853, -129.3179) -> (224.4853, -143.3229)
  line L357 (224.4853, -143.3229) -> (210.4803, -143.3229)
  line L358 (210.4803, -143.3229) -> (210.4803, -129.3179)
  line L359 (210.4803, -129.3179) -> (224.4853, -143.3229) construction
  line L360 (224.4853, -129.3179) -> (210.4803, -143.3229) construction
  line L361 (191.4303, -129.3179) -> (205.4353, -129.3179)
  line L362 (205.4353, -129.3179) -> (205.4353, -143.3229)
  line L363 (205.4353, -143.3229) -> (191.4303, -143.3229)
  line L364 (191.4303, -143.3229) -> (191.4303, -129.3179)
  line L365 (191.4303, -129.3179) -> (205.4353, -143.3229) construction
  line L366 (205.4353, -129.3179) -> (191.4303, -143.3229) construction
  line L367 (172.3803, -129.3179) -> (186.3853, -129.3179)
  line L368 (186.3853, -129.3179) -> (186.3853, -143.3229)
  line L369 (186.3853, -143.3229) -> (172.3803, -143.3229)
  line L370 (172.3803, -143.3229) -> (172.3803, -129.3179)
  line L371 (172.3803, -129.3179) -> (186.3853, -143.3229) construction
  line L372 (186.3853, -129.3179) -> (172.3803, -143.3229) construction
  line L373 (153.3303, -129.3179) -> (167.3353, -129.3179)
  line L374 (167.3353, -129.3179) -> (167.3353, -143.3229)
  line L375 (167.3353, -143.3229) -> (153.3303, -143.3229)
  line L376 (153.3303, -143.3229) -> (153.3303, -129.3179)
  line L377 (153.3303, -129.3179) -> (167.3353, -143.3229) construction
  line L378 (167.3353, -129.3179) -> (153.3303, -143.3229) construction
  line L379 (134.2803, -129.3179) -> (148.2853, -129.3179)
  line L380 (148.2853, -129.3179) -> (148.2853, -143.3229)
  line L381 (148.2853, -143.3229) -> (134.2803, -143.3229)
  line L382 (134.2803, -143.3229) -> (134.2803, -129.3179)
  line L383 (134.2803, -129.3179) -> (148.2853, -143.3229) construction
  line L384 (148.2853, -129.3179) -> (134.2803, -143.3229) construction
  line L385 (181.3976, -148.3679) -> (195.4026, -148.3679)
  line L386 (195.4026, -148.3679) -> (195.4026, -162.3729)
  line L387 (195.4026, -162.3729) -> (181.3976, -162.3729)
  line L388 (181.3976, -162.3729) -> (181.3976, -148.3679)
  line L389 (181.3976, -148.3679) -> (195.4026, -162.3729) construction
  line L390 (195.4026, -148.3679) -> (181.3976, -162.3729) construction
  line L391 (115.2303, -129.3179) -> (129.2353, -129.3179)
  line L392 (129.2353, -129.3179) -> (129.2353, -143.3229)
  line L393 (129.2353, -143.3229) -> (115.2303, -143.3229)
  line L394 (115.2303, -143.3229) -> (115.2303, -129.3179)
  line L395 (115.2303, -129.3179) -> (129.2353, -143.3229) construction
  line L396 (129.2353, -129.3179) -> (115.2303, -143.3229) construction
  line L397 (96.1803, -129.3179) -> (110.1853, -129.3179)
  line L398 (110.1853, -129.3179) -> (110.1853, -143.3229)
  line L399 (110.1853, -143.3229) -> (96.1803, -143.3229)
  line L400 (96.1803, -143.3229) -> (96.1803, -129.3179)
  line L401 (96.1803, -129.3179) -> (110.1853, -143.3229) construction
  line L402 (110.1853, -129.3179) -> (96.1803, -143.3229) construction
  line L403 (77.1303, -129.3179) -> (91.1353, -129.3179)
  line L404 (91.1353, -129.3179) -> (91.1353, -143.3229)
  line L405 (91.1353, -143.3229) -> (77.1303, -143.3229)
  line L406 (77.1303, -143.3229) -> (77.1303, -129.3179)
  line L407 (77.1303, -129.3179) -> (91.1353, -143.3229) construction
  line L408 (91.1353, -129.3179) -> (77.1303, -143.3229) construction
  line L409 (50.9683, -129.3179) -> (64.9733, -129.3179)
  line L410 (64.9733, -129.3179) -> (64.9733, -143.3229)
  line L411 (64.9733, -143.3229) -> (50.9683, -143.3229)
  line L412 (50.9683, -143.3229) -> (50.9683, -129.3179)
  line L413 (50.9683, -129.3179) -> (64.9733, -143.3229) construction
  line L414 (64.9733, -129.3179) -> (50.9683, -143.3229) construction
  line L415 (59.8583, -148.3679) -> (73.8633, -148.3679)
  line L416 (73.8633, -148.3679) -> (73.8633, -162.3729)
  line L417 (73.8633, -162.3729) -> (59.8583, -162.3729)
  line L418 (59.8583, -162.3729) -> (59.8583, -148.3679)
  line L419 (59.8583, -148.3679) -> (73.8633, -162.3729) construction
  line L420 (73.8633, -148.3679) -> (59.8583, -162.3729) construction
  line L421 (83.7343, -148.3679) -> (97.7393, -148.3679)
  line L422 (97.7393, -148.3679) -> (97.7393, -162.3729)
  line L423 (97.7393, -162.3729) -> (83.7343, -162.3729)
  line L424 (83.7343, -162.3729) -> (83.7343, -148.3679)
  line L425 (83.7343, -148.3679) -> (97.7393, -162.3729) construction
  line L426 (97.7393, -148.3679) -> (83.7343, -162.3729) construction
  line L427 (45.2568, -91.4679) -> (47.2568, -91.4679)
  line L428 (47.2568, -91.4679) -> (47.2568, -89.9679)
  line L429 (47.2568, -89.9679) -> (49.2568, -89.9679)
  line L430 (49.2568, -89.9679) -> (49.2568, -91.4679)
  line L431 (49.2568, -91.4679) -> (51.2568, -91.4679)
  line L432 (51.2568, -91.4679) -> (51.2568, -103.9679)
  line L433 (51.2568, -103.9679) -> (45.2568, -103.9679)
  line L434 (45.2568, -103.9679) -> (45.2568, -91.4679)
  line L435 (69.2568, -91.4679) -> (71.2568, -91.4679)
  line L436 (71.2568, -91.4679) -> (71.2568, -89.9679)
  line L437 (71.2568, -89.9679) -> (73.2568, -89.9679)
  line L438 (73.2568, -89.9679) -> (73.2568, -91.4679)
  line L439 (73.2568, -91.4679) -> (75.2568, -91.4679)
  line L440 (75.2568, -91.4679) -> (75.2568, -103.9679)
  line L441 (75.2568, -103.9679) -> (69.2568, -103.9679)
  line L442 (69.2568, -103.9679) -> (69.2568, -91.4679)
  line L443 (118.6501, -148.6179) -> (120.6501, -148.6179)
  line L444 (120.6501, -148.6179) -> (120.6501, -147.1179)
  line L445 (120.6501, -147.1179) -> (122.6501, -147.1179)
  line L446 (122.6501, -147.1179) -> (122.6501, -148.6179)
  line L447 (122.6501, -148.6179) -> (124.6501, -148.6179)
  line L448 (124.6501, -148.6179) -> (124.6501, -161.1179)
  line L449 (124.6501, -161.1179) -> (118.6501, -161.1179)
  line L450 (118.6501, -161.1179) -> (118.6501, -148.6179)
  line L451 (252.1501, -148.6179) -> (254.1501, -148.6179)
  line L452 (254.1501, -148.6179) -> (254.1501, -147.1179)
  line L453 (254.1501, -147.1179) -> (256.1501, -147.1179)
  line L454 (256.1501, -147.1179) -> (256.1501, -148.6179)
  line L455 (256.1501, -148.6179) -> (258.1501, -148.6179)
  line L456 (258.1501, -148.6179) -> (258.1501, -161.1179)
  line L457 (258.1501, -161.1179) -> (252.1501, -161.1179)
  line L458 (252.1501, -161.1179) -> (252.1501, -148.6179)
  circle A338 centre (45, -64.8616) radius 3.25
  circle A339 centre (45, -127) radius 3.25
  circle A340 centre (155, -64.8616) radius 3.25
  circle A341 centre (265, -160) radius 3.25
  circle A342 centre (155, -160) radius 3.25
  line L459 (269.4528, -40) -> (269.4528, -60.9161)
  line L460 (269.4528, -60.9161) -> (260.1818, -60.9161)
  line L461 (260.1818, -60.9161) -> (260.1818, -88.7954)
  line L462 (260.1818, -88.7954) -> (269.5798, -88.7954)
  line L463 (269.5798, -88.7954) -> (269.5798, -107.8454)
  line L464 (269.5798, -107.8454) -> (274.6598, -107.8454)
  line L465 (274.6598, -107.8454) -> (274.6598, -126.6954)
  line L466 (274.6598, -126.6954) -> (265.0048, -126.6954)
  line L467 (265.0048, -126.6954) -> (265.0048, -148.2602)
  line L468 (265.0048, -148.2602) -> (272.0064, -148.2602)
  line L469 (272.0064, -148.2602) -> (272.0064, -165)
  line L470 (272.0064, -165) -> (40, -165)
  line L471 (40, -165) -> (40, -40)
  line L472 (40, -40) -> (269.4528, -40)
  line L473 (-1718.9722, -136.3204) -> (-1718.9722, -148.1602) construction
  line L474 (-1718.9722, -148.1602) -> (-1718.9722, -160) construction
  line L475 (265.1048, -148.1602) -> (264.2819, -148.1602) construction
  line L476 (265, -160) -> (265, -148.1602) construction
  line L477 (265, -160) -> (276.8398, -160) construction
  line L478 (272.1064, -148.1602) -> (274.6328, -148.1602) construction
  line L479 (274.6328, -148.1602) -> (274.6328, -136.3204) construction
  point P0 (0, 0)
  point P1 (46.7679, -124.2729)
  point P2 (46.1423, -123.9574)
  dimension "d0" = 2
  dimension "d1" = 2
  dimension "d2" = 2
  dimension "d3" = 2
  dimension "d5" = 14.005
  dimension "d6" = 14.005
  dimension "d7" = 14.005
  dimension "d8" = 14.005
  dimension "d9" = 14.005
  dimension "d10" = 14.005
  dimension "d11" = 14.005
  dimension "d12" = 14.005
  dimension "d13" = 14.005
  dimension "d14" = 14.005
  dimension "d15" = 14.005
  dimension "d16" = 14.005
  dimension "d17" = 14.005
  dimension "d18" = 14.005
  dimension "d19" = 14.005
  dimension "d20" = 14.005
  dimension "d21" = 14.005
  dimension "d22" = 14.005
  dimension "d23" = 14.005
  dimension "d24" = 14.005
  dimension "d25" = 14.005
  dimension "d26" = 14.005
  dimension "d27" = 14.005
  dimension "d28" = 14.005
  dimension "d29" = 14.005
  dimension "d30" = 14.005
  dimension "d31" = 14.005
  dimension "d32" = 14.005
  dimension "d33" = 14.005
  dimension "d34" = 14.005
  dimension "d35" = 14.005
  dimension "d36" = 14.005
  dimension "d37" = 14.005
  dimension "d38" = 14.005
  dimension "d39" = 14.005
  dimension "d40" = 14.005
  dimension "d41" = 14.005
  dimension "d42" = 14.005
  dimension "d43" = 14.005
  dimension "d44" = 14.005
  dimension "d45" = 14.005
  dimension "d46" = 14.005
  dimension "d47" = 14.005
  dimension "d48" = 14.005
  dimension "d49" = 14.005
  dimension "d50" = 14.005
  dimension "d51" = 14.005
  dimension "d52" = 14.005